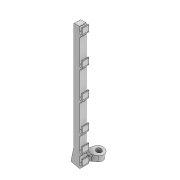
# Autodesk Inventor part: Wasserlevel_Kabelhalter_210403
Saved by Autodesk Inventor 2020 (Build 240168000, 168)
## iProperties
Created: 2020-10-31
Part Number: Wasserlevel_Kabelhalter_210403
Material: Generisch
Document SubType Name: Modeling
Designer: uhlma
Density: 1 g/cm^3
Appearance: Vorgabe
Author: uhlma
Autodesk Inventor part; units mm, degrees
ref_plane "YZ Plane" through (0, 0, 0) normal (1, 0, 0) x (0, 1, 0)
ref_plane "XZ Plane" through (0, 0, 0) normal (0, 1, 0) x (-1, 0, 0)
ref_plane "XY Plane" through (0, 0, 0) normal (0, 0, 1) x (1, 0, 0)
sketch "Skizze1" plane through (0, 0, 0) normal (0, 0, 1) x (1, 0, 0)
  circle A0 centre (4, 2.411) radius 0.575 construction
  arc A1 (3.675, 3.0026) -> (4.675, 2.411) centre (4, 2.411) ccw
  line L0 (4.675, 5.911) -> (4.675, 2.411)
  line L1 (4, 2.411) -> (4, 6.6743) construction
  line L2 (0, 5) -> (0, 0)
  line L3 (3.675, 0) -> (5.043, 1.368)
  arc A2 (5.043, 1.368) -> (5.475, 2.411) centre (4, 2.411) ccw
  line L4 (3.675, 5) -> (3.675, 3.0026)
  line L5 (5.475, 2.411) -> (5.475, 5.911)
  line L6 (3.675, 5) -> (0, 5)
  line L7 (0, 0) -> (3.675, 0)
  circle A3 centre (4, 2.411) radius 1.475 construction
  line L8 (4.675, 5.911) -> (5.475, 5.911)
  dimension "d0" = 1.15
  dimension "d5" = 3.5
  dimension "d6" = 4
  dimension "d7" = 45
  dimension "d9" = 0.8
  dimension "d13" = 0.1
  dimension "d15" = 1
  dimension "d21" = 5
  constraints: 18 end point, 4 centre point, 4 point on circle, 4 tangent, 4 vertical, 3 coincident, 1 horizontal, 1 horizontal alignment, 1 parallel, 1 perpendicular, 1 vertical alignment
  measures "d0" diameter of A0
  measures "d5" vertical distance of L5.end A0.centre
  measures "d6" distance from line of L2 A0.centre
  measures "d7" angle of L3 L2
  measures "d9" radial gap between concentric circles of A1 A3
  measures "d13" radial gap between concentric circles of A0 A1
  measures "d15" distance between parallel lines of L0 L4
  measures "d21" distance between parallel lines of L6 L7
extrude "Extrusion1" add sketch "Skizze1" along normal mid plane 4
pattern_linear "Rechteckige Anordnung3" count 2 spacing 7 along (0, 1, 0) of "Extrusion1"
pattern_linear "Rechteckige Anordnung4" count 5 spacing 18 along (0, 1, 0) of "Extrusion1"
sketch "Skizze6" plane through (0, 0, 2) normal (0, 0, 1) x (1, 0, 0)
  line L0 (0, 5) -> (0, 0) projected
  line L1 (0, 0) -> (0, 77.911)
  line L2 (0, 77.911) -> (3.675, 77.911)
  line L3 (3.675, 75.0026) -> (3.675, 77) projected
  line L4 (3.675, 77.911) -> (3.675, 77)
  line L5 (3.675, 72) -> (5.043, 73.368) projected
  line L6 (3.675, 57.0026) -> (3.675, 59) projected
  line L7 (3.675, 72) -> (3.675, 59)
  line L8 (3.675, 54) -> (5.043, 55.368) projected
  line L9 (3.675, 41) -> (3.675, 39.0026) projected
  line L10 (3.675, 54) -> (3.675, 41)
  line L11 (3.675, 36) -> (5.043, 37.368) projected
  line L12 (3.675, 36) -> (3.675, 23)
  line L13 (3.675, 18) -> (5.043, 19.368) projected
  line L14 (3.675, 18) -> (3.675, 12)
  line L15 (3.675, 7) -> (5.043, 8.368) projected
  line L16 (3.675, 3.0026) -> (3.675, 5) projected
  line L17 (3.675, 7) -> (3.675, 5)
  line L18 (3.675, 5) -> (0, 5) projected
  line L19 (0, 7) -> (3.675, 7) projected
  line L20 (3.675, 12) -> (0, 12) projected
  line L21 (0, 18) -> (3.675, 18) projected
  line L22 (3.675, 23) -> (0, 23) projected
  line L23 (0, 36) -> (3.675, 36) projected
  line L24 (3.675, 41) -> (0, 41) projected
  line L25 (0, 54) -> (3.675, 54) projected
  line L26 (3.675, 59) -> (0, 59) projected
  line L27 (0, 72) -> (3.675, 72) projected
  line L28 (3.675, 77) -> (0, 77) projected
  point P0 (0, 5)
  constraints: 14 end point, 4 vertical, 1 collinear, 1 horizontal, 1 perpendicular, 3 other
extrude "Extrusion6" add sketch "Skizze6" against normal up to surface (4 mm away)
fillet "Rundung4" radius 0.2 20 edges at (3.675, 3.0026, 0) (4.675, 5.911, 0) (5.475, 5.911, 0) (5.475, 12.911, 0) (4.675, 12.911, 0) (3.675, 10.0026, 0) (3.675, 21.0026, 0) (4.675, 23.911, 0) (5.475, 23.911, 0) (3.675, 39.0026, 0) (4.675, 41.911, 0) (5.475, 41.911, 0) (3.675, 57.0026, 0) (4.675, 59.911, 0) (5.475, 59.911, 0) (3.675, 75.0026, 0) (4.675, 77.911, 0) (5.475, 77.911, 0) (3.675, 77.911, 0) (0, 77.911, 0)
fillet "Rundung4" radius 1 5 edges at (3.675, 72, 0) (3.675, 54, 0) (3.675, 36, 0) (3.675, 18, 0) (3.675, 7, 0)
sketch "Skizze5" plane through (0, 0, 2) normal (0, 0, 1) x (1, 0, 0)
  line L0 (-8.2168, 2.5277) -> (3.675, 0)
  line L1 (-8.2168, 2.5277) -> (-8.2168, 0)
  line L2 (3.675, 0) -> (0, 0) projected
  line L3 (-8.2168, 0) -> (3.675, 0)
  dimension "d38" = 12
  constraints: 6 end point, 1 coincident, 1 perpendicular, 1 vertical
  measures "d38" angle of L2 L0
extrude "Extrusion5" cut sketch "Skizze5" against normal through all
sketch "Skizze4" plane through (0.0349, 0.7737, 0) normal (0.2079117, 0.9781476, 0) x (-0.9781476, 0.2079117, 0)
  line L0 (0.0356, -2) -> (0.0356, 2) projected
  line L1 (0.0356, 2) -> (-3.7215, 2) projected
  circle A0 centre (-2.9644, -10) radius 1.65
  circle A1 centre (-2.9644, -10) radius 3.25
  line L2 (-3.7215, -2) -> (0.0356, -2) projected
  line L3 (-4.7751, -2) -> (-3.7215, -2) projected
  line L4 (0.0356, -2) -> (16.0303, -2) projected
  line L5 (2.0356, -2) -> (2.0356, 2)
  line L6 (16.0303, 2) -> (0.0356, 2) projected
  line L7 (-3.7215, 2) -> (-4.7751, 2) projected
  line L8 (-3.7215, -2) -> (-2.7215, -2)
  line L9 (-2.7215, -2) -> (-2.7215, -5)
  line L10 (-2.7215, -5) -> (-5.331, -7.7725)
  line L11 (2.0356, 2) -> (0.0356, 2)
  line L12 (2.0356, -2) -> (0.2163, -10.6676)
  dimension "d41" = 3.3
  dimension "d57" = 1.6
  dimension "d59" = 3
  dimension "d61" = 2
  dimension "d72" = 8
  dimension "d73" = 1
  dimension "d74" = 3
  constraints: 12 end point, 2 centre point, 2 point on circle, 2 point on line, 2 tangent, 1 coincident, 1 collinear, 1 perpendicular, 1 vertical
  measures "d41" diameter of A0
  measures "d57" radial gap between concentric circles of A1 A0
  measures "d59" horizontal distance of L0.start A0.centre
  measures "d61" distance between parallel lines of L0 L5
  measures "d72" distance from line of L2 A0.centre
  measures "d73" distance of L2.start L8.end
  measures "d74" distance of L8.end L9.end
extrude "Extrusion4" add sketch "Skizze4" along normal blind 4
sketch "Skizze7" plane through (0.8665, 4.6863, 0) normal (0.2079117, 0.9781476, 0) x (0.9781476, -0.2079117, 0)
  line L0 (-0.8859, 2) -> (-16.0303, 2) projected
  line L1 (-0.8859, 2) -> (-2.0356, 2)
  line L2 (-2.0356, 2) -> (-2.0356, -2)
  line L3 (-2.0356, -2) -> (-0.8859, -2)
  line L4 (-0.8859, -2) -> (-0.8859, 2)
  point P0 (-2.0356, 2)
  constraints: 8 end point, 2 parallel, 1 horizontal, 1 perpendicular
extrude "Extrusion7" add sketch "Skizze7" against normal up to surface surface through (0, 12, 0) normal (-1, 0, 0)
fillet "Rundung8" radius 3.5 2 edges at (0, 10.4006, 0) (1.2019, 4.615, -2)
fillet "Rundung9" radius 2 1 edges at (3.1164, 2.1818, -5)
